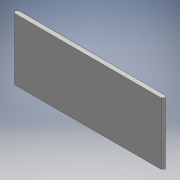
# Autodesk Inventor part: Pieza2
Saved by Autodesk Inventor 2016 (Build 200138000, 138)
## iProperties
Created: 2016-10-17
Part Number: Pieza2
Material: Genérico
Document SubType Name: Modeling
Designer: Roberto
Density: 1 g/cm^3
Appearance: Valor por defecto
Author: Roberto
Autodesk Inventor part; units mm, degrees
ref_plane "YZ Plane" through (0, 0, 0) normal (1, 0, 0) x (0, 1, 0)
ref_plane "XZ Plane" through (0, 0, 0) normal (0, 1, 0) x (-1, 0, 0)
ref_plane "XY Plane" through (0, 0, 0) normal (0, 0, 1) x (1, 0, 0)
sketch "Boceto1" plane through (0, 0, 0) normal (0, 1, 0) x (-1, 0, 0)
  line L0 (0, 0) -> (0, -7)
  line L1 (0, -7) -> (16.6, -7)
  line L2 (16.6, -7) -> (16.6, 0)
  line L3 (16.6, 0) -> (0, 0)
  dimension "d0" = 7
  dimension "d1" = 16.6
  dimension "d2" = 7
  constraints: 8 end point, 1 horizontal, 1 perpendicular, 1 vertical
  measures "d0" distance of L0.start L0.end
  measures "d1" distance of L0.end L1.end
  measures "d2" distance of L1.end L2.end
extrude "Extrusión1" add sketch "Boceto1" along normal blind 0.5
sketch "Boceto2" plane through (-16.6, 0, 0) normal (0, 0, 1) x (1, 0, 0)
  line L0 (16.6, 0.5) -> (16.6, 0)
  line L1 (16.6, 0.5) -> (16.85, 0.25)
  line L2 (16.85, 0.25) -> (16.6, 0)
  line L3 (0, 0) -> (16.6, 0) projected
  line L4 (16.6, 0) -> (16.6, 0.5) projected
  line L5 (0, 0.5) -> (16.6, 0.5) projected
  line L6 (0, 0) -> (0, 0.5) projected
  line L7 (0, 0.5) -> (0, 0)
  line L8 (0, 0.5) -> (-0.25, 0.25)
  line L9 (-0.25, 0.25) -> (0, 0)
  line L10 (0, 0) -> (0, 0.5)
  constraints: 14 end point, 1 perpendicular, 1 vertical
extrude "Extrusión2" add sketch "Boceto2" against normal blind 7 contours L1 L2 L0 | L6 L9 L8
sketch "Boceto3" plane through (0, 0.5, 0) normal (0, 1, 0) x (1, 0, 0)
  line L0 (-16.6, 7) -> (-16.6, 0) projected
  line L1 (0, 0) -> (0, 7) projected
  circle A0 centre (-8.3, 3.5) radius 0.4
  circle A1 centre (-14.1, 3.5) radius 0.4
  circle A2 centre (-2.5, 3.5) radius 0.4
  dimension "d8" = 0.8
  dimension "d9" = 0.8
  constraints: 3 centre point
  measures "d8" diameter of A0
  measures "d9" diameter of A1
extrude "Extrusión3" cut sketch "Boceto3" against normal blind 0.35
